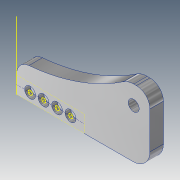
# Autodesk Inventor part: XbearingBracket
Saved by Autodesk Inventor 2019 (Build 230136000, 136)
## iProperties
Created: 2018-10-14
Part Number: XbearingBracket
Material: Aluminum 6061
Document SubType Name: Modeling
Designer: LillaHunden
Density: 2.7 g/cm^3
Appearance: Aluminum - Flat
Mass: 56.2677 g
Surface Area: 71.9907 cm^2
Volume: 20.8399 cm^3
Author: LillaHunden
Autodesk Inventor part; units mm, degrees
ref_plane "YZ Plane" through (0, 0, 0) normal (1, 0, 0) x (0, 1, 0)
ref_plane "XZ Plane" through (0, 0, 0) normal (0, 1, 0) x (-1, 0, 0)
ref_plane "XY Plane" through (0, 0, 0) normal (0, 0, 1) x (1, 0, 0)
sketch "Sketch1" plane through (0, 0, 0) normal (0, 0, 1) x (1, 0, 0)
  line L0 (0, 0) -> (79.0225, 0)
  line L1 (79.0225, 0) -> (79.0225, 40)
  line L2 (79.0225, 40) -> (0, 40)
  line L3 (0, 40) -> (0, 0)
  dimension "d33" = 40
  constraints: 8 end point, 2 parallel, 1 horizontal, 1 perpendicular
  measures "d33" distance of L0.end L1.end
extrude "Extrusion1" add sketch "Sketch1" along normal blind 8
sketch "Sketch2" plane through (0, 0, 0) normal (0, 0, -1) x (-1, 0, 0)
  circle A0 centre (-69.4131, 28.9577) radius 2.5 construction
  circle A1 centre (-69.4131, 28.9577) radius 4.765
  point P0 (0, 0)
  dimension "d2" = 9.53
  constraints: 1 centre point, 1 coincident
  measures "d2" diameter of A1
extrude "Extrusion2" cut sketch "Sketch2" against normal blind 3.3
sketch "Sketch3" plane through (69.4131, 28.9577, 3.3) normal (0, 0, -1) x (-1, 0, 0)
  circle A0 centre (0, 0) radius 3.25
  point P0 (69.4131, -28.9577)
  dimension "d5" = 6.5
  constraints: 1 centre point
  measures "d5" diameter of A0
extrude "Extrusion3" cut sketch "Sketch3" against normal through all
sketch "Sketch4" plane through (0, 0, 8) normal (0, 0, 1) x (1, 0, 0)
  line L0 (0, 0) -> (40, 0) construction
  line L1 (40, 0) -> (40, 10) construction
  line L2 (0, 10) -> (40, 10) construction
  line L3 (0, 0) -> (0, 10) construction
  line L4 (40, 5) -> (0, 5) construction
  line L5 (0, 40) -> (0, 0) projected
  circle A0 centre (16, 5) radius 1.2295 projected
  circle A1 centre (32, 5) radius 1.2295 projected
  circle A2 centre (24, 5) radius 1.2295 projected
  circle A3 centre (8, 5) radius 1.2295 projected
  point P0 (32, 5)
  point P1 (24, 5)
  point P2 (16, 5)
  point P3 (8, 5)
  dimension "d8" = 8
  dimension "d9" = 8
  dimension "d10" = 8
  dimension "d11" = 8
  constraints: 5 point on line, 2 end point, 1 horizontal, 1 midpoint
  measures "d8" distance from line of L3 point (8, 5)
  measures "d9" distance from line of L1 point (32, 5)
  measures "d10" distance of point (24, 5) point (32, 5)
  measures "d11" distance of point (8, 5) point (16, 5)
sketch "Sketch6" plane through (0, 0, 8) normal (0, 0, 1) x (1, 0, 0)
  point P0 (32, 5)
  point P1 (24, 5)
  point P2 (16, 5)
  point P3 (8, 5)
hole "Hole2" at (32, 5, 8) at (24, 5, 8) at (16, 5, 8) at (8, 5, 8) direction (0, 0, -1) diameter 3.2 depth 8 counterbore diameter 6.5 counterbore depth 3.4
sketch "Sketch7" plane through (0, 0, 8) normal (0, 0, 1) x (1, 0, 0)
  circle A0 centre (16, 5) radius 1.2295 construction
  circle A1 centre (32, 5) radius 1.2295 construction
  circle A2 centre (24, 5) radius 1.2295 construction
  circle A3 centre (8, 5) radius 1.2295 construction
  line L0 (0, 0) -> (40, 0) construction
  line L1 (40, 0) -> (40, 10) construction
  line L2 (0, 10) -> (40, 10) construction
  line L3 (0, 0) -> (0, 10) construction
  circle A4 centre (69.4131, 28.9577) radius 3.25 projected
  circle A5 centre (69.4131, 28.9577) radius 11.0423
  line L4 (79.0225, 40) -> (0, 40) projected
  arc A6 (0, 18.0455) -> (63.2734, 38.1358) centre (-3.1135, 137.5348) ccw
  line L5 (0, 10) -> (0, 18.0455)
  line L6 (0, 40) -> (0, 0) projected
  line L7 (69.4131, 40) -> (0, 40)
  line L8 (0, 40) -> (0, 18.0455)
  constraints: 6 end point, 5 point on circle, 2 centre point, 2 point on line, 1 coincident, 1 collinear, 1 horizontal, 1 tangent
extrude "Extrusion4" cut sketch "Sketch7" against normal through all contours A5 A6 L6 L4
fillet "Fillet2" radius 10 1 edges at (79.0225, 0, 4)
fillet "Fillet3" radius 8 2 edges at (79.0225, 40, 4) (0, 18.0455, 4)
equation "\"d9\" = d8"
equation "\"d10\" = d9"
equation "\"d11\" = d8"
body "Solid1"
